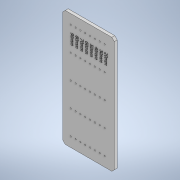
# Autodesk Inventor part: A-01
Saved by Autodesk Inventor 2022 (Build 260153000, 153)
## iProperties
Created: 2021-10-10
Part Number: A-01
Material: Generic
Document SubType Name: Modeling
Designer: kfcs7
Density: 1 g/cm^3
Appearance: Default
Author: kfcs7
Autodesk Inventor part; units mm, degrees
(part 1 of 2)
ref_plane "YZ Plane" through (0, 0, 0) normal (1, 0, 0) x (0, 1, 0)
ref_plane "XZ Plane" through (0, 0, 0) normal (0, 1, 0) x (-1, 0, 0)
ref_plane "XY Plane" through (0, 0, 0) normal (0, 0, 1) x (1, 0, 0)
sketch "Sketch1" plane through (0, 0, 0) normal (0, 0, 1) x (1, 0, 0)
  line L0 (14.5, -5) -> (14.5, -245) construction
  line L1 (14.5, -5) -> (0, -5) construction
  line L2 (0, -5) -> (0, -245) construction
  line L3 (0, -245) -> (14.5, -245) construction
  circle A0 centre (6.5, -25) radius 3.25 construction
  circle A1 centre (6.5, -75) radius 3.25 construction
  circle A2 centre (6.5, -125) radius 3.25 construction
  circle A3 centre (6.5, -175) radius 3.25 construction
  circle A4 centre (6.5, -225) radius 3.25 construction
  line L4 (26.5, -5) -> (-80, -5)
  line L5 (-80, -5) -> (-80, -245)
  line L6 (-80, -245) -> (26.5, -245)
  line L7 (26.5, -245) -> (26.5, -5)
  point P0 (0, 0)
  dimension "d6" = 20
  dimension "d9" = 80
  constraints: 8 end point, 2 collinear, 2 parallel, 1 horizontal, 1 perpendicular
  measures "d6" distance from line of L7 A0.centre
  measures "d9" distance between parallel lines of L2 L5
extrude "Extrusion1" add sketch "Sketch1" along normal blind 6
sketch "Sketch3" plane through (0, 0, 6) normal (0, 0, 1) x (1, 0, 0)
  line L0 (14.5, -5) -> (14.5, -245) construction
  line L1 (14.5, -5) -> (0, -5) construction
  line L2 (0, -5) -> (0, -245) construction
  line L3 (0, -245) -> (14.5, -245) construction
  circle A0 centre (6.5, -25) radius 3.25 construction
  circle A1 centre (6.5, -75) radius 3.25 construction
  circle A2 centre (6.5, -125) radius 3.25 construction
  circle A3 centre (6.5, -175) radius 3.25 construction
  circle A4 centre (6.5, -225) radius 3.25 construction
  circle A5 centre (6.5, -25) radius 1.25
  circle A6 centre (6.5, -75) radius 1.25
  circle A7 centre (6.5, -125) radius 1.25
  circle A8 centre (6.5, -175) radius 1.25
  circle A9 centre (6.5, -225) radius 1.25
  point P0 (0, 0)
  dimension "d10" = 2.5
  dimension "d11" = 2.5
  dimension "d12" = 2.5
  dimension "d13" = 2.5
  dimension "d14" = 2.5
  constraints: 5 centre point, 5 coincident
  measures "d10" diameter of A5
  measures "d11" diameter of A6
  measures "d12" diameter of A7
  measures "d13" diameter of A8
  measures "d14" diameter of A9
extrude "Extrusion2" cut sketch "Sketch3" against normal through all
chamfer "Chamfer1" distance 5 angle 45 4 edges at (26.5, -5, 3) (-80, -5, 3) (-80, -245, 3) (26.5, -245, 3)
pattern_linear "Rectangular Pattern1" count 8 spacing 10 along (-1, 0, 0) of "Extrusion2"
sketch "Sketch4" plane through (0, 0, 6) normal (0, 0, 1) x (1, 0, 0)
  circle A0 centre (6.5, -75) radius 1.25 construction
  circle A1 centre (6.5, -175) radius 1.25 construction
  circle A2 centre (6.5, -125) radius 1.25 construction
  circle A3 centre (6.5, -25) radius 1.25 construction
  circle A4 centre (6.5, -225) radius 1.25 construction
  line L0 (-80, -10) -> (-80, -240) construction
  line L1 (-75, -245) -> (21.5, -245) construction
  line L2 (26.5, -240) -> (26.5, -10) construction
  line L3 (21.5, -5) -> (-75, -5) construction
  circle A5 centre (6.5, -25) radius 1.25 construction
  circle A6 centre (6.5, -75) radius 1.25 construction
  line L4 (6.5, -25) -> (6.5, -75) construction
  line L5 (26.5, -240) -> (21.5, -245) construction
  line L6 (21.5, -5) -> (26.5, -10) construction
  line L7 (-80, -10) -> (-75, -5) construction
  line L8 (-75, -245) -> (-80, -240) construction
  circle A7 centre (-63.5, -75) radius 1.25 construction
  circle A8 centre (-63.5, -225) radius 1.25 construction
  circle A9 centre (-63.5, -25) radius 1.25 construction
  circle A10 centre (-63.5, -125) radius 1.25 construction
  circle A11 centre (-63.5, -175) radius 1.25 construction
  circle A12 centre (-53.5, -75) radius 1.25 construction
  circle A13 centre (-53.5, -225) radius 1.25 construction
  circle A14 centre (-53.5, -25) radius 1.25 construction
  circle A15 centre (-53.5, -125) radius 1.25 construction
  circle A16 centre (-53.5, -175) radius 1.25 construction
  circle A17 centre (-43.5, -75) radius 1.25 construction
  circle A18 centre (-43.5, -225) radius 1.25 construction
  circle A19 centre (-43.5, -25) radius 1.25 construction
  circle A20 centre (-43.5, -125) radius 1.25 construction
  circle A21 centre (-43.5, -175) radius 1.25 construction
  circle A22 centre (-33.5, -75) radius 1.25 construction
  circle A23 centre (-33.5, -225) radius 1.25 construction
  circle A24 centre (-33.5, -25) radius 1.25 construction
  circle A25 centre (-33.5, -125) radius 1.25 construction
  circle A26 centre (-33.5, -175) radius 1.25 construction
  circle A27 centre (-23.5, -75) radius 1.25 construction
  circle A28 centre (-23.5, -225) radius 1.25 construction
  circle A29 centre (-23.5, -25) radius 1.25 construction
  circle A30 centre (-23.5, -125) radius 1.25 construction
  circle A31 centre (-23.5, -175) radius 1.25 construction
  circle A32 centre (-13.5, -75) radius 1.25 construction
  circle A33 centre (-13.5, -225) radius 1.25 construction
  circle A34 centre (-13.5, -25) radius 1.25 construction
  circle A35 centre (-13.5, -125) radius 1.25 construction
  circle A36 centre (-13.5, -175) radius 1.25 construction
  circle A37 centre (-3.5, -75) radius 1.25 construction
  circle A38 centre (-3.5, -225) radius 1.25 construction
  circle A39 centre (-3.5, -25) radius 1.25 construction
  circle A40 centre (-3.5, -125) radius 1.25 construction
  circle A41 centre (-3.5, -175) radius 1.25 construction
  line L9 (26.5, -240) -> (21.5, -245) construction
  line L10 (26.5, -240) -> (26.5, -10) construction
  line L11 (21.5, -5) -> (26.5, -10) construction
  line L12 (21.5, -5) -> (-75, -5) construction
  line L13 (-80, -10) -> (-75, -5) construction
  line L14 (-80, -10) -> (-80, -240) construction
  line L15 (-75, -245) -> (-80, -240) construction
  line L16 (-75, -245) -> (21.5, -245) construction
  circle A42 centre (6.5, -75) radius 1.25 construction
  circle A43 centre (6.5, -175) radius 1.25 construction
  circle A44 centre (6.5, -125) radius 1.25 construction
  circle A45 centre (6.5, -25) radius 1.25 construction
  circle A46 centre (6.5, -225) radius 1.25 construction
  circle A47 centre (-3.5, -25) radius 1.25 construction
  line L17 (-3.5, -25) -> (-3.5, -75) construction
  circle A48 centre (-13.5, -75) radius 1.25 construction
  line L18 (-13.5, -25) -> (-13.5, -75) construction
  circle A49 centre (-23.5, -75) radius 1.25 construction
  circle A50 centre (-23.5, -25) radius 1.25 construction
  line L19 (-23.5, -75) -> (-23.5, -25) construction
  circle A51 centre (-33.5, -25) radius 1.25 construction
  circle A52 centre (-33.5, -75) radius 1.25 construction
  line L20 (-33.5, -25) -> (-33.5, -75) construction
  circle A53 centre (-43.5, -75) radius 1.25 construction
  circle A54 centre (-43.5, -25) radius 1.25 construction
  line L21 (-43.5, -75) -> (-43.5, -25) construction
  circle A55 centre (-53.5, -25) radius 1.25 construction
  circle A56 centre (-53.5, -75) radius 1.25 construction
  line L22 (-53.5, -25) -> (-53.5, -75) construction
  circle A57 centre (-63.5, -25) radius 1.25 construction
  circle A58 centre (-63.5, -75) radius 1.25 construction
  line L23 (-63.5, -25) -> (-63.5, -75) construction
  line L24 (6.5, -42.5851) -> (6.5, -38.8233)
  line L25 (6.5, -38.8233) -> (7.3651, -38.8233)
  spline S0 degree 2 poles (7.3651, -38.8233) (7.7457, -39.2286) (8.4526, -39.9503) (8.8332, -40.2964) knots 0 0 0 1 2 2 2
  spline S1 degree 2 poles (8.8332, -40.2964) (9.5994, -40.9934) (10.5189, -41.5025) (11.0083, -41.5025) knots 0 0 0 1 2 2 2
  spline S2 degree 2 poles (11.0083, -41.5025) (11.2653, -41.5025) (11.6509, -41.3443) (11.7745, -41.201) knots 0 0 0 1 2 2 2
  spline S3 degree 2 poles (11.7745, -41.201) (11.8981, -41.0576) (12.0216, -40.6819) (12.0216, -40.4545) knots 0 0 0 1 2 2 2
  spline S4 degree 2 poles (12.0216, -40.4545) (12.0216, -40.237) (11.9129, -39.7921) (11.8288, -39.5895) knots 0 0 0 1 2 2 2
  spline S5 degree 2 poles (11.8288, -39.5895) (11.7596, -39.4165) (11.5619, -39.0951) (11.4927, -38.9963) knots 0 0 0 1 2 2 2
  line L26 (11.4927, -38.9963) -> (11.4927, -38.9518)
  line L27 (11.4927, -38.9518) -> (12.3627, -38.9518)
  spline S6 degree 2 poles (12.3627, -38.9518) (12.4863, -39.2039) (12.7285, -40.1085) (12.7285, -40.5139) knots 0 0 0 1 2 2 2
  spline S7 degree 2 poles (12.7285, -40.5139) (12.7285, -41.369) (11.8239, -42.333) (11.0528, -42.333) knots 0 0 0 1 2 2 2
  spline S8 degree 2 poles (11.0528, -42.333) (10.6919, -42.333) (10.0888, -42.1649) (9.8318, -42.0166) knots 0 0 0 1 2 2 2
  spline S9 degree 2 poles (9.8318, -42.0166) (9.5648, -41.8683) (9.0408, -41.4382) (8.7887, -41.201) knots 0 0 0 1 2 2 2
  spline S10 degree 2 poles (8.7887, -41.201) (8.3686, -40.8154) (7.4689, -39.8712) (7.2069, -39.5895) knots 0 0 0 1 2 2 2
  line L28 (7.2069, -39.5895) -> (7.2069, -42.5851)
  line L29 (7.2069, -42.5851) -> (6.5, -42.5851)
  spline S11 degree 2 poles (9.55, -47.1972) (7.9088, -47.1972) (6.3715, -46.2431) (6.3715, -45.2495) knots 0 0 0 1 2 2 2
  spline S12 degree 2 poles (6.3715, -45.2495) (6.3715, -44.2411) (7.9385, -43.2969) (9.5451, -43.2969) knots 0 0 0 1 2 2 2
  spline S13 degree 2 poles (9.5451, -43.2969) (11.1961, -43.2969) (12.7236, -44.251) (12.7236, -45.2495) knots 0 0 0 1 2 2 2
  spline S14 degree 2 poles (12.7236, -45.2495) (12.7236, -46.253) (11.1417, -47.1972) (9.55, -47.1972) knots 0 0 0 1 2 2 2
  spline S15 degree 2 poles (7.6913, -46.1492) (7.9929, -46.2678) (8.9222, -46.3667) (9.55, -46.3667) knots 0 0 0 1 2 2 2
  spline S16 degree 2 poles (9.55, -46.3667) (10.1778, -46.3667) (11.1022, -46.2678) (11.4136, -46.1442) knots 0 0 0 1 2 2 2
  spline S17 degree 2 poles (11.4136, -46.1442) (11.725, -46.0207) (12.0464, -45.5906) (12.0464, -45.2495) knots 0 0 0 1 2 2 2
  spline S18 degree 2 poles (12.0464, -45.2495) (12.0464, -44.9084) (11.725, -44.4685) (11.4037, -44.34) knots 0 0 0 1 2 2 2
  spline S19 degree 2 poles (11.4037, -44.34) (11.0923, -44.2164) (10.1432, -44.1274) (9.5451, -44.1274) knots 0 0 0 1 2 2 2
  spline S20 degree 2 poles (9.5451, -44.1274) (8.9024, -44.1274) (8.0423, -44.2065) (7.7062, -44.335) knots 0 0 0 1 2 2 2
  spline S21 degree 2 poles (7.7062, -44.335) (7.3898, -44.4536) (7.0487, -44.8936) (7.0487, -45.2495) knots 0 0 0 1 2 2 2
  spline S22 degree 2 poles (7.0487, -45.2495) (7.0487, -45.5857) (7.37, -46.0256) (7.6913, -46.1492) knots 0 0 0 1 2 2 2
  line L30 (6.5, -53.2823) -> (9.1496, -53.2823)
  spline S23 degree 2 poles (9.1496, -53.2823) (9.466, -53.2823) (10.0048, -53.2329) (10.1531, -53.1538) knots 0 0 0 1 2 2 2
  spline S24 degree 2 poles (10.1531, -53.1538) (10.3162, -53.0747) (10.4744, -52.7732) (10.4744, -52.5112) knots 0 0 0 1 2 2 2
  spline S25 degree 2 poles (10.4744, -52.5112) (10.4744, -52.2739) (10.1827, -51.7301) (9.9059, -51.4434) knots 0 0 0 1 2 2 2
  spline S26 degree 2 poles (9.9059, -51.4434) (9.8367, -51.4484) (9.6439, -51.4583) (9.5154, -51.4583) knots 0 0 0 1 2 2 2
  line L31 (9.5154, -51.4583) -> (6.5, -51.4583)
  line L32 (6.5, -51.4583) -> (6.5, -50.6871)
  line L33 (6.5, -50.6871) -> (9.1496, -50.6871)
  spline S27 degree 2 poles (9.1496, -50.6871) (9.466, -50.6871) (10.0048, -50.6377) (10.1531, -50.5586) knots 0 0 0 1 2 2 2
  spline S28 degree 2 poles (10.1531, -50.5586) (10.3162, -50.4795) (10.4744, -50.178) (10.4744, -49.916) knots 0 0 0 1 2 2 2
  spline S29 degree 2 poles (10.4744, -49.916) (10.4744, -49.6688) (10.163, -49.1201) (9.9207, -48.863) knots 0 0 0 1 2 2 2
  line L34 (9.9207, -48.863) -> (6.5, -48.863)
  line L35 (6.5, -48.863) -> (6.5, -48.0919)
  line L36 (6.5, -48.0919) -> (11.0775, -48.0919)
  line L37 (11.0775, -48.0919) -> (11.0775, -48.863)
  line L38 (11.0775, -48.863) -> (10.5733, -48.863)
  spline S30 degree 2 poles (10.5733, -48.863) (10.8748, -49.1646) (11.206, -49.7578) (11.206, -50.1137) knots 0 0 0 1 2 2 2
  spline S31 degree 2 poles (11.206, -50.1137) (11.206, -50.519) (10.8353, -51.1468) (10.4151, -51.31) knots 0 0 0 1 2 2 2
  spline S32 degree 2 poles (10.4151, -51.31) (10.8056, -51.6609) (11.206, -52.3233) (11.206, -52.7089) knots 0 0 0 1 2 2 2
  spline S33 degree 2 poles (11.206, -52.7089) (11.206, -53.0055) (11.0231, -53.49) (10.8155, -53.6679) knots 0 0 0 1 2 2 2
  spline S34 degree 2 poles (10.8155, -53.6679) (10.6079, -53.8508) (9.985, -54.0535) (9.5154, -54.0535) knots 0 0 0 1 2 2 2
  line L39 (9.5154, -54.0535) -> (6.5, -54.0535)
  line L40 (6.5, -54.0535) -> (6.5, -53.2823)
  line L41 (6.5, -60.3265) -> (9.1496, -60.3265)
  spline S35 degree 2 poles (9.1496, -60.3265) (9.466, -60.3265) (10.0048, -60.2771) (10.1531, -60.198) knots 0 0 0 1 2 2 2
  spline S36 degree 2 poles (10.1531, -60.198) (10.3162, -60.1189) (10.4744, -59.8173) (10.4744, -59.5553) knots 0 0 0 1 2 2 2
  spline S37 degree 2 poles (10.4744, -59.5553) (10.4744, -59.3181) (10.1827, -58.7743) (9.9059, -58.4876) knots 0 0 0 1 2 2 2
  spline S38 degree 2 poles (9.9059, -58.4876) (9.8367, -58.4925) (9.6439, -58.5024) (9.5154, -58.5024) knots 0 0 0 1 2 2 2
  line L42 (9.5154, -58.5024) -> (6.5, -58.5024)
  line L43 (6.5, -58.5024) -> (6.5, -57.7313)
  line L44 (6.5, -57.7313) -> (9.1496, -57.7313)
  spline S39 degree 2 poles (9.1496, -57.7313) (9.466, -57.7313) (10.0048, -57.6818) (10.1531, -57.6028) knots 0 0 0 1 2 2 2
  spline S40 degree 2 poles (10.1531, -57.6028) (10.3162, -57.5237) (10.4744, -57.2221) (10.4744, -56.9601) knots 0 0 0 1 2 2 2
  spline S41 degree 2 poles (10.4744, -56.9601) (10.4744, -56.713) (10.163, -56.1643) (9.9207, -55.9072) knots 0 0 0 1 2 2 2
  line L45 (9.9207, -55.9072) -> (6.5, -55.9072)
  line L46 (6.5, -55.9072) -> (6.5, -55.1361)
  line L47 (6.5, -55.1361) -> (11.0775, -55.1361)
  line L48 (11.0775, -55.1361) -> (11.0775, -55.9072)
  line L49 (11.0775, -55.9072) -> (10.5733, -55.9072)
  spline S42 degree 2 poles (10.5733, -55.9072) (10.8748, -56.2088) (11.206, -56.8019) (11.206, -57.1579) knots 0 0 0 1 2 2 2
  spline S43 degree 2 poles (11.206, -57.1579) (11.206, -57.5632) (10.8353, -58.191) (10.4151, -58.3541) knots 0 0 0 1 2 2 2
  spline S44 degree 2 poles (10.4151, -58.3541) (10.8056, -58.7051) (11.206, -59.3675) (11.206, -59.7531) knots 0 0 0 1 2 2 2
  spline S45 degree 2 poles (11.206, -59.7531) (11.206, -60.0497) (11.0231, -60.5341) (10.8155, -60.7121) knots 0 0 0 1 2 2 2
  spline S46 degree 2 poles (10.8155, -60.7121) (10.6079, -60.895) (9.985, -61.0976) (9.5154, -61.0976) knots 0 0 0 1 2 2 2
  line L50 (9.5154, -61.0976) -> (6.5, -61.0976)
  line L51 (6.5, -61.0976) -> (6.5, -60.3265)
  spline S47 degree 2 poles (2.0216, -40.4694) (2.0216, -40.2469) (1.9129, -39.807) (1.8288, -39.5944) knots 0 0 0 1 2 2 2
  spline S48 degree 2 poles (1.8288, -39.5944) (1.7448, -39.3967) (1.5669, -39.105) (1.4878, -38.9913) knots 0 0 0 1 2 2 2
  line L52 (1.4878, -38.9913) -> (1.4878, -38.9419)
  line L53 (1.4878, -38.9419) -> (2.3528, -38.9419)
  spline S49 degree 2 poles (2.3528, -38.9419) (2.4962, -39.2088) (2.7285, -40.1233) (2.7285, -40.5336) knots 0 0 0 1 2 2 2
  spline S50 degree 2 poles (2.7285, -40.5336) (2.7285, -40.9489) (2.5605, -41.5668) (2.3825, -41.8189) knots 0 0 0 1 2 2 2
  spline S51 degree 2 poles (2.3825, -41.8189) (2.1897, -42.0858) (1.6311, -42.3626) (1.2554, -42.3626) knots 0 0 0 1 2 2 2
  spline S52 degree 2 poles (1.2554, -42.3626) (0.7512, -42.3626) (-0.01, -41.7002) (-0.1089, -41.2356) knots 0 0 0 1 2 2 2
  line L54 (-0.1089, -41.2356) -> (-0.1682, -41.2356)
  spline S53 degree 2 poles (-0.1682, -41.2356) (-0.2078, -41.4284) (-0.3857, -41.8683) (-0.5637, -42.0562) knots 0 0 0 1 2 2 2
  spline S54 degree 2 poles (-0.5637, -42.0562) (-0.7367, -42.244) (-1.2904, -42.4813) (-1.6908, -42.4813) knots 0 0 0 1 2 2 2
  spline S55 degree 2 poles (-1.6908, -42.4813) (-2.1011, -42.4813) (-2.7981, -42.1995) (-3.065, -41.9425) knots 0 0 0 1 2 2 2
  spline S56 degree 2 poles (-3.065, -41.9425) (-3.3418, -41.6755) (-3.6285, -40.9192) (-3.6285, -40.4397) knots 0 0 0 1 2 2 2
  spline S57 degree 2 poles (-3.6285, -40.4397) (-3.6285, -39.98) (-3.4061, -39.0803) (-3.2528, -38.7738) knots 0 0 0 1 2 2 2
  line L55 (-3.2528, -38.7738) -> (-2.3878, -38.7738)
  line L56 (-2.3878, -38.7738) -> (-2.3878, -38.8331)
  spline S58 degree 2 poles (-2.3878, -38.8331) (-2.5756, -39.0902) (-2.9216, -39.9602) (-2.9216, -40.3903) knots 0 0 0 1 2 2 2
  spline S59 degree 2 poles (-2.9216, -40.3903) (-2.9216, -40.6424) (-2.7635, -41.1466) (-2.5806, -41.3147) knots 0 0 0 1 2 2 2
  spline S60 degree 2 poles (-2.5806, -41.3147) (-2.3976, -41.4778) (-1.9626, -41.6508) (-1.6314, -41.6508) knots 0 0 0 1 2 2 2
  spline S61 degree 2 poles (-1.6314, -41.6508) (-1.3002, -41.6508) (-0.8702, -41.458) (-0.7466, -41.285) knots 0 0 0 1 2 2 2
  spline S62 degree 2 poles (-0.7466, -41.285) (-0.623, -41.112) (-0.5291, -40.6424) (-0.5291, -40.3656) knots 0 0 0 1 2 2 2
  line L57 (-0.5291, -40.3656) -> (-0.5291, -40.0195)
  line L58 (-0.5291, -40.0195) -> (0.1481, -40.0195)
  line L59 (0.1481, -40.0195) -> (0.1481, -40.2914)
  spline S63 degree 2 poles (0.1481, -40.2914) (0.1481, -40.8401) (0.6721, -41.5322) (1.1714, -41.5322) knots 0 0 0 1 2 2 2
  spline S64 degree 2 poles (1.1714, -41.5322) (1.4037, -41.5322) (1.7349, -41.3542) (1.8338, -41.2109) knots 0 0 0 1 2 2 2
  spline S65 degree 2 poles (1.8338, -41.2109) (1.9376, -41.0576) (2.0216, -40.6819) (2.0216, -40.4694) knots 0 0 0 1 2 2 2
  spline S66 degree 2 poles (-0.45, -47.1972) (-2.0912, -47.1972) (-3.6285, -46.2431) (-3.6285, -45.2495) knots 0 0 0 1 2 2 2
  spline S67 degree 2 poles (-3.6285, -45.2495) (-3.6285, -44.2411) (-2.0615, -43.2969) (-0.4549, -43.2969) knots 0 0 0 1 2 2 2
  spline S68 degree 2 poles (-0.4549, -43.2969) (1.1961, -43.2969) (2.7236, -44.251) (2.7236, -45.2495) knots 0 0 0 1 2 2 2
  spline S69 degree 2 poles (2.7236, -45.2495) (2.7236, -46.253) (1.1417, -47.1972) (-0.45, -47.1972) knots 0 0 0 1 2 2 2
  spline S70 degree 2 poles (-2.3087, -46.1492) (-2.0071, -46.2678) (-1.0778, -46.3667) (-0.45, -46.3667) knots 0 0 0 1 2 2 2
  spline S71 degree 2 poles (-0.45, -46.3667) (0.1778, -46.3667) (1.1022, -46.2678) (1.4136, -46.1442) knots 0 0 0 1 2 2 2
  spline S72 degree 2 poles (1.4136, -46.1442) (1.725, -46.0207) (2.0464, -45.5906) (2.0464, -45.2495) knots 0 0 0 1 2 2 2
  spline S73 degree 2 poles (2.0464, -45.2495) (2.0464, -44.9084) (1.725, -44.4685) (1.4037, -44.34) knots 0 0 0 1 2 2 2
  spline S74 degree 2 poles (1.4037, -44.34) (1.0923, -44.2164) (0.1432, -44.1274) (-0.4549, -44.1274) knots 0 0 0 1 2 2 2
  spline S75 degree 2 poles (-0.4549, -44.1274) (-1.0976, -44.1274) (-1.9577, -44.2065) (-2.2938, -44.335) knots 0 0 0 1 2 2 2
  spline S76 degree 2 poles (-2.2938, -44.335) (-2.6102, -44.4536) (-2.9513, -44.8936) (-2.9513, -45.2495) knots 0 0 0 1 2 2 2
  spline S77 degree 2 poles (-2.9513, -45.2495) (-2.9513, -45.5857) (-2.63, -46.0256) (-2.3087, -46.1492) knots 0 0 0 1 2 2 2
  line L60 (-3.5, -53.2823) -> (-0.8504, -53.2823)
  spline S78 degree 2 poles (-0.8504, -53.2823) (-0.534, -53.2823) (0.0048, -53.2329) (0.1531, -53.1538) knots 0 0 0 1 2 2 2
  spline S79 degree 2 poles (0.1531, -53.1538) (0.3162, -53.0747) (0.4744, -52.7732) (0.4744, -52.5112) knots 0 0 0 1 2 2 2
  spline S80 degree 2 poles (0.4744, -52.5112) (0.4744, -52.2739) (0.1827, -51.7301) (-0.0941, -51.4434) knots 0 0 0 1 2 2 2
  spline S81 degree 2 poles (-0.0941, -51.4434) (-0.1633, -51.4484) (-0.3561, -51.4583) (-0.4846, -51.4583) knots 0 0 0 1 2 2 2
  line L61 (-0.4846, -51.4583) -> (-3.5, -51.4583)
  line L62 (-3.5, -51.4583) -> (-3.5, -50.6871)
  line L63 (-3.5, -50.6871) -> (-0.8504, -50.6871)
  spline S82 degree 2 poles (-0.8504, -50.6871) (-0.534, -50.6871) (0.0048, -50.6377) (0.1531, -50.5586) knots 0 0 0 1 2 2 2
  spline S83 degree 2 poles (0.1531, -50.5586) (0.3162, -50.4795) (0.4744, -50.178) (0.4744, -49.916) knots 0 0 0 1 2 2 2
  spline S84 degree 2 poles (0.4744, -49.916) (0.4744, -49.6688) (0.163, -49.1201) (-0.0793, -48.863) knots 0 0 0 1 2 2 2
  line L64 (-0.0793, -48.863) -> (-3.5, -48.863)
  line L65 (-3.5, -48.863) -> (-3.5, -48.0919)
  line L66 (-3.5, -48.0919) -> (1.0775, -48.0919)
  line L67 (1.0775, -48.0919) -> (1.0775, -48.863)
  line L68 (1.0775, -48.863) -> (0.5733, -48.863)
  spline S85 degree 2 poles (0.5733, -48.863) (0.8748, -49.1646) (1.206, -49.7578) (1.206, -50.1137) knots 0 0 0 1 2 2 2
  spline S86 degree 2 poles (1.206, -50.1137) (1.206, -50.519) (0.8353, -51.1468) (0.4151, -51.31) knots 0 0 0 1 2 2 2
  spline S87 degree 2 poles (0.4151, -51.31) (0.8056, -51.6609) (1.206, -52.3233) (1.206, -52.7089) knots 0 0 0 1 2 2 2
  spline S88 degree 2 poles (1.206, -52.7089) (1.206, -53.0055) (1.0231, -53.49) (0.8155, -53.6679) knots 0 0 0 1 2 2 2
  spline S89 degree 2 poles (0.8155, -53.6679) (0.6079, -53.8508) (-0.015, -54.0535) (-0.4846, -54.0535) knots 0 0 0 1 2 2 2
  line L69 (-0.4846, -54.0535) -> (-3.5, -54.0535)
  line L70 (-3.5, -54.0535) -> (-3.5, -53.2823)
  line L71 (-3.5, -60.3265) -> (-0.8504, -60.3265)
  spline S90 degree 2 poles (-0.8504, -60.3265) (-0.534, -60.3265) (0.0048, -60.2771) (0.1531, -60.198) knots 0 0 0 1 2 2 2
  spline S91 degree 2 poles (0.1531, -60.198) (0.3162, -60.1189) (0.4744, -59.8173) (0.4744, -59.5553) knots 0 0 0 1 2 2 2
  spline S92 degree 2 poles (0.4744, -59.5553) (0.4744, -59.3181) (0.1827, -58.7743) (-0.0941, -58.4876) knots 0 0 0 1 2 2 2
  spline S93 degree 2 poles (-0.0941, -58.4876) (-0.1633, -58.4925) (-0.3561, -58.5024) (-0.4846, -58.5024) knots 0 0 0 1 2 2 2
  line L72 (-0.4846, -58.5024) -> (-3.5, -58.5024)
  line L73 (-3.5, -58.5024) -> (-3.5, -57.7313)
  line L74 (-3.5, -57.7313) -> (-0.8504, -57.7313)
  spline S94 degree 2 poles (-0.8504, -57.7313) (-0.534, -57.7313) (0.0048, -57.6818) (0.1531, -57.6028) knots 0 0 0 1 2 2 2
  spline S95 degree 2 poles (0.1531, -57.6028) (0.3162, -57.5237) (0.4744, -57.2221) (0.4744, -56.9601) knots 0 0 0 1 2 2 2
  spline S96 degree 2 poles (0.4744, -56.9601) (0.4744, -56.713) (0.163, -56.1643) (-0.0793, -55.9072) knots 0 0 0 1 2 2 2
  line L75 (-0.0793, -55.9072) -> (-3.5, -55.9072)
  line L76 (-3.5, -55.9072) -> (-3.5, -55.1361)
  line L77 (-3.5, -55.1361) -> (1.0775, -55.1361)
  line L78 (1.0775, -55.1361) -> (1.0775, -55.9072)
  line L79 (1.0775, -55.9072) -> (0.5733, -55.9072)
  spline S97 degree 2 poles (0.5733, -55.9072) (0.8748, -56.2088) (1.206, -56.8019) (1.206, -57.1579) knots 0 0 0 1 2 2 2
  spline S98 degree 2 poles (1.206, -57.1579) (1.206, -57.5632) (0.8353, -58.191) (0.4151, -58.3541) knots 0 0 0 1 2 2 2
  spline S99 degree 2 poles (0.4151, -58.3541) (0.8056, -58.7051) (1.206, -59.3675) (1.206, -59.7531) knots 0 0 0 1 2 2 2
  spline S100 degree 2 poles (1.206, -59.7531) (1.206, -60.0497) (1.0231, -60.5341) (0.8155, -60.7121) knots 0 0 0 1 2 2 2
  spline S101 degree 2 poles (0.8155, -60.7121) (0.6079, -60.895) (-0.015, -61.0976) (-0.4846, -61.0976) knots 0 0 0 1 2 2 2
  line L80 (-0.4846, -61.0976) -> (-3.5, -61.0976)
  line L81 (-3.5, -61.0976) -> (-3.5, -60.3265)
  line L82 (-11.4041, -42.7482) -> (-11.4041, -42.0216)
  line L83 (-11.4041, -42.0216) -> (-13.5, -42.0216)
  line L84 (-13.5, -42.0216) -> (-13.5, -41.2356)
  line L85 (-13.5, -41.2356) -> (-11.4041, -41.2356)
  line L86 (-11.4041, -41.2356) -> (-11.4041, -38.5415)
  line L87 (-11.4041, -38.5415) -> (-10.5439, -38.5415)
  line L88 (-10.5439, -38.5415) -> (-7.4, -41.2702)
  line L89 (-7.4, -41.2702) -> (-7.4, -42.0216)
  line L90 (-7.4, -42.0216) -> (-10.7466, -42.0216)
  line L91 (-10.7466, -42.0216) -> (-10.7466, -42.7482)
  line L92 (-10.7466, -42.7482) -> (-11.4041, -42.7482)
  line L93 (-10.7466, -41.2356) -> (-8.3639, -41.2356)
  line L94 (-8.3639, -41.2356) -> (-10.7466, -39.1841)
  line L95 (-10.7466, -39.1841) -> (-10.7466, -41.2356)
  spline S102 degree 2 poles (-10.45, -47.1972) (-12.0912, -47.1972) (-13.6285, -46.2431) (-13.6285, -45.2495) knots 0 0 0 1 2 2 2
  spline S103 degree 2 poles (-13.6285, -45.2495) (-13.6285, -44.2411) (-12.0615, -43.2969) (-10.4549, -43.2969) knots 0 0 0 1 2 2 2
  spline S104 degree 2 poles (-10.4549, -43.2969) (-8.8039, -43.2969) (-7.2764, -44.251) (-7.2764, -45.2495) knots 0 0 0 1 2 2 2
  spline S105 degree 2 poles (-7.2764, -45.2495) (-7.2764, -46.253) (-8.8583, -47.1972) (-10.45, -47.1972) knots 0 0 0 1 2 2 2
  spline S106 degree 2 poles (-12.3087, -46.1492) (-12.0071, -46.2678) (-11.0778, -46.3667) (-10.45, -46.3667) knots 0 0 0 1 2 2 2
  spline S107 degree 2 poles (-10.45, -46.3667) (-9.8222, -46.3667) (-8.8978, -46.2678) (-8.5864, -46.1442) knots 0 0 0 1 2 2 2
  spline S108 degree 2 poles (-8.5864, -46.1442) (-8.275, -46.0207) (-7.9536, -45.5906) (-7.9536, -45.2495) knots 0 0 0 1 2 2 2
  spline S109 degree 2 poles (-7.9536, -45.2495) (-7.9536, -44.9084) (-8.275, -44.4685) (-8.5963, -44.34) knots 0 0 0 1 2 2 2
  spline S110 degree 2 poles (-8.5963, -44.34) (-8.9077, -44.2164) (-9.8568, -44.1274) (-10.4549, -44.1274) knots 0 0 0 1 2 2 2
  spline S111 degree 2 poles (-10.4549, -44.1274) (-11.0976, -44.1274) (-11.9577, -44.2065) (-12.2938, -44.335) knots 0 0 0 1 2 2 2
  spline S112 degree 2 poles (-12.2938, -44.335) (-12.6102, -44.4536) (-12.9513, -44.8936) (-12.9513, -45.2495) knots 0 0 0 1 2 2 2
  spline S113 degree 2 poles (-12.9513, -45.2495) (-12.9513, -45.5857) (-12.63, -46.0256) (-12.3087, -46.1492) knots 0 0 0 1 2 2 2
  line L96 (-13.5, -53.2823) -> (-10.8504, -53.2823)
  spline S114 degree 2 poles (-10.8504, -53.2823) (-10.534, -53.2823) (-9.9952, -53.2329) (-9.8469, -53.1538) knots 0 0 0 1 2 2 2
  spline S115 degree 2 poles (-9.8469, -53.1538) (-9.6838, -53.0747) (-9.5256, -52.7732) (-9.5256, -52.5112) knots 0 0 0 1 2 2 2
  spline S116 degree 2 poles (-9.5256, -52.5112) (-9.5256, -52.2739) (-9.8173, -51.7301) (-10.0941, -51.4434) knots 0 0 0 1 2 2 2
  spline S117 degree 2 poles (-10.0941, -51.4434) (-10.1633, -51.4484) (-10.3561, -51.4583) (-10.4846, -51.4583) knots 0 0 0 1 2 2 2
  line L97 (-10.4846, -51.4583) -> (-13.5, -51.4583)
  line L98 (-13.5, -51.4583) -> (-13.5, -50.6871)
  line L99 (-13.5, -50.6871) -> (-10.8504, -50.6871)
  spline S118 degree 2 poles (-10.8504, -50.6871) (-10.534, -50.6871) (-9.9952, -50.6377) (-9.8469, -50.5586) knots 0 0 0 1 2 2 2
  spline S119 degree 2 poles (-9.8469, -50.5586) (-9.6838, -50.4795) (-9.5256, -50.178) (-9.5256, -49.916) knots 0 0 0 1 2 2 2
  spline S120 degree 2 poles (-9.5256, -49.916) (-9.5256, -49.6688) (-9.837, -49.1201) (-10.0793, -48.863) knots 0 0 0 1 2 2 2
  line L100 (-10.0793, -48.863) -> (-13.5, -48.863)
  line L101 (-13.5, -48.863) -> (-13.5, -48.0919)
  line L102 (-13.5, -48.0919) -> (-8.9225, -48.0919)
  line L103 (-8.9225, -48.0919) -> (-8.9225, -48.863)
  line L104 (-8.9225, -48.863) -> (-9.4267, -48.863)
  spline S121 degree 2 poles (-9.4267, -48.863) (-9.1252, -49.1646) (-8.794, -49.7578) (-8.794, -50.1137) knots 0 0 0 1 2 2 2
  spline S122 degree 2 poles (-8.794, -50.1137) (-8.794, -50.519) (-9.1647, -51.1468) (-9.5849, -51.31) knots 0 0 0 1 2 2 2
  spline S123 degree 2 poles (-9.5849, -51.31) (-9.1944, -51.6609) (-8.794, -52.3233) (-8.794, -52.7089) knots 0 0 0 1 2 2 2
  spline S124 degree 2 poles (-8.794, -52.7089) (-8.794, -53.0055) (-8.9769, -53.49) (-9.1845, -53.6679) knots 0 0 0 1 2 2 2
  spline S125 degree 2 poles (-9.1845, -53.6679) (-9.3921, -53.8508) (-10.015, -54.0535) (-10.4846, -54.0535) knots 0 0 0 1 2 2 2
  line L105 (-10.4846, -54.0535) -> (-13.5, -54.0535)
  line L106 (-13.5, -54.0535) -> (-13.5, -53.2823)
  line L107 (-13.5, -60.3265) -> (-10.8504, -60.3265)
  spline S126 degree 2 poles (-10.8504, -60.3265) (-10.534, -60.3265) (-9.9952, -60.2771) (-9.8469, -60.198) knots 0 0 0 1 2 2 2
  spline S127 degree 2 poles (-9.8469, -60.198) (-9.6838, -60.1189) (-9.5256, -59.8173) (-9.5256, -59.5553) knots 0 0 0 1 2 2 2
  spline S128 degree 2 poles (-9.5256, -59.5553) (-9.5256, -59.3181) (-9.8173, -58.7743) (-10.0941, -58.4876) knots 0 0 0 1 2 2 2
  spline S129 degree 2 poles (-10.0941, -58.4876) (-10.1633, -58.4925) (-10.3561, -58.5024) (-10.4846, -58.5024) knots 0 0 0 1 2 2 2
  line L108 (-10.4846, -58.5024) -> (-13.5, -58.5024)
  line L109 (-13.5, -58.5024) -> (-13.5, -57.7313)
  line L110 (-13.5, -57.7313) -> (-10.8504, -57.7313)
  spline S130 degree 2 poles (-10.8504, -57.7313) (-10.534, -57.7313) (-9.9952, -57.6818) (-9.8469, -57.6028) knots 0 0 0 1 2 2 2
  spline S131 degree 2 poles (-9.8469, -57.6028) (-9.6838, -57.5237) (-9.5256, -57.2221) (-9.5256, -56.9601) knots 0 0 0 1 2 2 2
  spline S132 degree 2 poles (-9.5256, -56.9601) (-9.5256, -56.713) (-9.837, -56.1643) (-10.0793, -55.9072) knots 0 0 0 1 2 2 2
  line L111 (-10.0793, -55.9072) -> (-13.5, -55.9072)
  line L112 (-13.5, -55.9072) -> (-13.5, -55.1361)
  line L113 (-13.5, -55.1361) -> (-8.9225, -55.1361)
  line L114 (-8.9225, -55.1361) -> (-8.9225, -55.9072)
  line L115 (-8.9225, -55.9072) -> (-9.4267, -55.9072)
  spline S133 degree 2 poles (-9.4267, -55.9072) (-9.1252, -56.2088) (-8.794, -56.8019) (-8.794, -57.1579) knots 0 0 0 1 2 2 2
  spline S134 degree 2 poles (-8.794, -57.1579) (-8.794, -57.5632) (-9.1647, -58.191) (-9.5849, -58.3541) knots 0 0 0 1 2 2 2
  spline S135 degree 2 poles (-9.5849, -58.3541) (-9.1944, -58.7051) (-8.794, -59.3675) (-8.794, -59.7531) knots 0 0 0 1 2 2 2
  spline S136 degree 2 poles (-8.794, -59.7531) (-8.794, -60.0497) (-8.9769, -60.5341) (-9.1845, -60.7121) knots 0 0 0 1 2 2 2
  spline S137 degree 2 poles (-9.1845, -60.7121) (-9.3921, -60.895) (-10.015, -61.0976) (-10.4846, -61.0976) knots 0 0 0 1 2 2 2
  line L116 (-10.4846, -61.0976) -> (-13.5, -61.0976)
  line L117 (-13.5, -61.0976) -> (-13.5, -60.3265)
  spline S138 degree 2 poles (-21.5622, -42.5208) (-22.0022, -42.5208) (-22.7536, -42.2391) (-23.0304, -41.982) knots 0 0 0 1 2 2 2
  spline S139 degree 2 poles (-23.0304, -41.982) (-23.3072, -41.725) (-23.6285, -40.9588) (-23.6285, -40.4842) knots 0 0 0 1 2 2 2
  spline S140 degree 2 poles (-23.6285, -40.4842) (-23.6285, -40.0492) (-23.4357, -39.1989) (-23.2825, -38.8875) knots 0 0 0 1 2 2 2
  line L118 (-23.2825, -38.8875) -> (-22.4174, -38.8875)
  line L119 (-22.4174, -38.8875) -> (-22.4174, -38.9468)
  spline S141 degree 2 poles (-22.4174, -38.9468) (-22.4866, -39.0408) (-22.6646, -39.3917) (-22.7437, -39.6043) knots 0 0 0 1 2 2 2
  spline S142 degree 2 poles (-22.7437, -39.6043) (-22.8277, -39.8465) (-22.9216, -40.2469) (-22.9216, -40.499) knots 0 0 0 1 2 2 2
  spline S143 degree 2 poles (-22.9216, -40.499) (-22.9216, -40.7462) (-22.7437, -41.2109) (-22.5509, -41.3789) knots 0 0 0 1 2 2 2
  spline S144 degree 2 poles (-22.5509, -41.3789) (-22.368, -41.5322) (-21.8835, -41.6904) (-21.5573, -41.6904) knots 0 0 0 1 2 2 2
  spline S145 degree 2 poles (-21.5573, -41.6904) (-21.231, -41.6904) (-20.8158, -41.5124) (-20.6774, -41.3443) knots 0 0 0 1 2 2 2
  spline S146 degree 2 poles (-20.6774, -41.3443) (-20.5241, -41.1713) (-20.3956, -40.6572) (-20.3956, -40.3458) knots 0 0 0 1 2 2 2
  spline S147 degree 2 poles (-20.3956, -40.3458) (-20.3956, -40.0096) (-20.4994, -39.3423) (-20.5439, -39.1396) knots 0 0 0 1 2 2 2
  line L120 (-20.5439, -39.1396) -> (-17.4, -39.1396)
  line L121 (-17.4, -39.1396) -> (-17.4, -42.4862)
  line L122 (-17.4, -42.4862) -> (-18.1168, -42.4862)
  line L123 (-18.1168, -42.4862) -> (-18.1168, -39.9256)
  line L124 (-18.1168, -39.9256) -> (-19.7431, -39.9256)
  spline S148 degree 2 poles (-19.7431, -39.9256) (-19.7233, -40.0739) (-19.7085, -40.3606) (-19.7085, -40.4793) knots 0 0 0 1 2 2 2
  spline S149 degree 2 poles (-19.7085, -40.4793) (-19.7085, -40.9489) (-19.8618, -41.5964) (-20.0891, -41.893) knots 0 0 0 1 2 2 2
  spline S150 degree 2 poles (-20.0891, -41.893) (-20.3165, -42.1946) (-21.0086, -42.5208) (-21.5622, -42.5208) knots 0 0 0 1 2 2 2
  spline S151 degree 2 poles (-20.45, -47.1972) (-22.0912, -47.1972) (-23.6285, -46.2431) (-23.6285, -45.2495) knots 0 0 0 1 2 2 2
  spline S152 degree 2 poles (-23.6285, -45.2495) (-23.6285, -44.2411) (-22.0615, -43.2969) (-20.4549, -43.2969) knots 0 0 0 1 2 2 2
  spline S153 degree 2 poles (-20.4549, -43.2969) (-18.8039, -43.2969) (-17.2764, -44.251) (-17.2764, -45.2495) knots 0 0 0 1 2 2 2
  spline S154 degree 2 poles (-17.2764, -45.2495) (-17.2764, -46.253) (-18.8583, -47.1972) (-20.45, -47.1972) knots 0 0 0 1 2 2 2
  spline S155 degree 2 poles (-22.3087, -46.1492) (-22.0071, -46.2678) (-21.0778, -46.3667) (-20.45, -46.3667) knots 0 0 0 1 2 2 2
  spline S156 degree 2 poles (-20.45, -46.3667) (-19.8222, -46.3667) (-18.8978, -46.2678) (-18.5864, -46.1442) knots 0 0 0 1 2 2 2
  spline S157 degree 2 poles (-18.5864, -46.1442) (-18.275, -46.0207) (-17.9536, -45.5906) (-17.9536, -45.2495) knots 0 0 0 1 2 2 2
  spline S158 degree 2 poles (-17.9536, -45.2495) (-17.9536, -44.9084) (-18.275, -44.4685) (-18.5963, -44.34) knots 0 0 0 1 2 2 2
  spline S159 degree 2 poles (-18.5963, -44.34) (-18.9077, -44.2164) (-19.8568, -44.1274) (-20.4549, -44.1274) knots 0 0 0 1 2 2 2
  spline S160 degree 2 poles (-20.4549, -44.1274) (-21.0976, -44.1274) (-21.9577, -44.2065) (-22.2938, -44.335) knots 0 0 0 1 2 2 2
  spline S161 degree 2 poles (-22.2938, -44.335) (-22.6102, -44.4536) (-22.9513, -44.8936) (-22.9513, -45.2495) knots 0 0 0 1 2 2 2
  spline S162 degree 2 poles (-22.9513, -45.2495) (-22.9513, -45.5857) (-22.63, -46.0256) (-22.3087, -46.1492) knots 0 0 0 1 2 2 2
  line L125 (-23.5, -53.2823) -> (-20.8504, -53.2823)
  spline S163 degree 2 poles (-20.8504, -53.2823) (-20.534, -53.2823) (-19.9952, -53.2329) (-19.8469, -53.1538) knots 0 0 0 1 2 2 2
  spline S164 degree 2 poles (-19.8469, -53.1538) (-19.6838, -53.0747) (-19.5256, -52.7732) (-19.5256, -52.5112) knots 0 0 0 1 2 2 2
  spline S165 degree 2 poles (-19.5256, -52.5112) (-19.5256, -52.2739) (-19.8173, -51.7301) (-20.0941, -51.4434) knots 0 0 0 1 2 2 2
  spline S166 degree 2 poles (-20.0941, -51.4434) (-20.1633, -51.4484) (-20.3561, -51.4583) (-20.4846, -51.4583) knots 0 0 0 1 2 2 2
  line L126 (-20.4846, -51.4583) -> (-23.5, -51.4583)
  line L127 (-23.5, -51.4583) -> (-23.5, -50.6871)
  line L128 (-23.5, -50.6871) -> (-20.8504, -50.6871)
  spline S167 degree 2 poles (-20.8504, -50.6871) (-20.534, -50.6871) (-19.9952, -50.6377) (-19.8469, -50.5586) knots 0 0 0 1 2 2 2
  spline S168 degree 2 poles (-19.8469, -50.5586) (-19.6838, -50.4795) (-19.5256, -50.178) (-19.5256, -49.916) knots 0 0 0 1 2 2 2
  spline S169 degree 2 poles (-19.5256, -49.916) (-19.5256, -49.6688) (-19.837, -49.1201) (-20.0793, -48.863) knots 0 0 0 1 2 2 2
  line L129 (-20.0793, -48.863) -> (-23.5, -48.863)
  line L130 (-23.5, -48.863) -> (-23.5, -48.0919)
  line L131 (-23.5, -48.0919) -> (-18.9225, -48.0919)
  line L132 (-18.9225, -48.0919) -> (-18.9225, -48.863)
  line L133 (-18.9225, -48.863) -> (-19.4267, -48.863)
  spline S170 degree 2 poles (-19.4267, -48.863) (-19.1252, -49.1646) (-18.794, -49.7578) (-18.794, -50.1137) knots 0 0 0 1 2 2 2
  spline S171 degree 2 poles (-18.794, -50.1137) (-18.794, -50.519) (-19.1647, -51.1468) (-19.5849, -51.31) knots 0 0 0 1 2 2 2
  spline S172 degree 2 poles (-19.5849, -51.31) (-19.1944, -51.6609) (-18.794, -52.3233) (-18.794, -52.7089) knots 0 0 0 1 2 2 2
  spline S173 degree 2 poles (-18.794, -52.7089) (-18.794, -53.0055) (-18.9769, -53.49) (-19.1845, -53.6679) knots 0 0 0 1 2 2 2
  spline S174 degree 2 poles (-19.1845, -53.6679) (-19.3921, -53.8508) (-20.015, -54.0535) (-20.4846, -54.0535) knots 0 0 0 1 2 2 2
  line L134 (-20.4846, -54.0535) -> (-23.5, -54.0535)
  line L135 (-23.5, -54.0535) -> (-23.5, -53.2823)
  line L136 (-23.5, -60.3265) -> (-20.8504, -60.3265)
  spline S175 degree 2 poles (-20.8504, -60.3265) (-20.534, -60.3265) (-19.9952, -60.2771) (-19.8469, -60.198) knots 0 0 0 1 2 2 2
  spline S176 degree 2 poles (-19.8469, -60.198) (-19.6838, -60.1189) (-19.5256, -59.8173) (-19.5256, -59.5553) knots 0 0 0 1 2 2 2
  spline S177 degree 2 poles (-19.5256, -59.5553) (-19.5256, -59.3181) (-19.8173, -58.7743) (-20.0941, -58.4876) knots 0 0 0 1 2 2 2
  spline S178 degree 2 poles (-20.0941, -58.4876) (-20.1633, -58.4925) (-20.3561, -58.5024) (-20.4846, -58.5024) knots 0 0 0 1 2 2 2
  line L137 (-20.4846, -58.5024) -> (-23.5, -58.5024)
  line L138 (-23.5, -58.5024) -> (-23.5, -57.7313)
  line L139 (-23.5, -57.7313) -> (-20.8504, -57.7313)
  spline S179 degree 2 poles (-20.8504, -57.7313) (-20.534, -57.7313) (-19.9952, -57.6818) (-19.8469, -57.6028) knots 0 0 0 1 2 2 2
  spline S180 degree 2 poles (-19.8469, -57.6028) (-19.6838, -57.5237) (-19.5256, -57.2221) (-19.5256, -56.9601) knots 0 0 0 1 2 2 2
  spline S181 degree 2 poles (-19.5256, -56.9601) (-19.5256, -56.713) (-19.837, -56.1643) (-20.0793, -55.9072) knots 0 0 0 1 2 2 2
  line L140 (-20.0793, -55.9072) -> (-23.5, -55.9072)
  line L141 (-23.5, -55.9072) -> (-23.5, -55.1361)
  line L142 (-23.5, -55.1361) -> (-18.9225, -55.1361)
  line L143 (-18.9225, -55.1361) -> (-18.9225, -55.9072)
  line L144 (-18.9225, -55.9072) -> (-19.4267, -55.9072)
  spline S182 degree 2 poles (-19.4267, -55.9072) (-19.1252, -56.2088) (-18.794, -56.8019) (-18.794, -57.1579) knots 0 0 0 1 2 2 2
  spline S183 degree 2 poles (-18.794, -57.1579) (-18.794, -57.5632) (-19.1647, -58.191) (-19.5849, -58.3541) knots 0 0 0 1 2 2 2
  spline S184 degree 2 poles (-19.5849, -58.3541) (-19.1944, -58.7051) (-18.794, -59.3675) (-18.794, -59.7531) knots 0 0 0 1 2 2 2
  spline S185 degree 2 poles (-18.794, -59.7531) (-18.794, -60.0497) (-18.9769, -60.5341) (-19.1845, -60.7121) knots 0 0 0 1 2 2 2
  spline S186 degree 2 poles (-19.1845, -60.7121) (-19.3921, -60.895) (-20.015, -61.0976) (-20.4846, -61.0976) knots 0 0 0 1 2 2 2
  line L145 (-20.4846, -61.0976) -> (-23.5, -61.0976)
  line L146 (-23.5, -61.0976) -> (-23.5, -60.3265)
  spline S187 degree 2 poles (-31.5227, -42.679) (-31.9923, -42.679) (-32.7882, -42.3676) (-33.0551, -42.1056) knots 0 0 0 1 2 2 2
  spline S188 degree 2 poles (-33.0551, -42.1056) (-33.3369, -41.8337) (-33.6285, -41.1515) (-33.6285, -40.7412) knots 0 0 0 1 2 2 2
  spline S189 degree 2 poles (-33.6285, -40.7412) (-33.6285, -40.331) (-33.3517, -39.6537) (-33.0749, -39.3967) knots 0 0 0 1 2 2 2
  spline S190 degree 2 poles (-33.0749, -39.3967) (-32.7437, -39.0803) (-31.6314, -38.7244) (-30.8207, -38.7244) knots 0 0 0 1 2 2 2
  spline S191 degree 2 poles (-30.8207, -38.7244) (-30.0249, -38.7244) (-28.7446, -39.0506) (-28.27, -39.3917) knots 0 0 0 1 2 2 2
  spline S192 degree 2 poles (-28.27, -39.3917) (-27.8053, -39.7229) (-27.2863, -40.7709) (-27.2863, -41.458) knots 0 0 0 1 2 2 2
  spline S193 degree 2 poles (-27.2863, -41.458) (-27.2863, -41.6607) (-27.3259, -42.0166) (-27.3703, -42.1501) knots 0 0 0 1 2 2 2
  line L147 (-27.3703, -42.1501) -> (-28.1563, -42.1501)
  line L148 (-28.1563, -42.1501) -> (-28.1563, -42.1155)
  spline S194 degree 2 poles (-28.1563, -42.1155) (-28.097, -42.0018) (-27.9932, -41.5865) (-27.9932, -41.3493) knots 0 0 0 1 2 2 2
  spline S195 degree 2 poles (-27.9932, -41.3493) (-27.9932, -40.588) (-29.0214, -39.6537) (-30.0298, -39.5647) knots 0 0 0 1 2 2 2
  spline S196 degree 2 poles (-30.0298, -39.5647) (-29.8271, -39.8564) (-29.6047, -40.4694) (-29.6047, -40.8352) knots 0 0 0 1 2 2 2
  spline S197 degree 2 poles (-29.6047, -40.8352) (-29.6047, -41.1911) (-29.7481, -41.725) (-29.9656, -42.0166) knots 0 0 0 1 2 2 2
  spline S198 degree 2 poles (-29.9656, -42.0166) (-30.2177, -42.3528) (-30.9987, -42.679) (-31.5227, -42.679) knots 0 0 0 1 2 2 2
  spline S199 degree 2 poles (-31.5573, -41.8485) (-31.1816, -41.8485) (-30.6724, -41.6508) (-30.4945, -41.4333) knots 0 0 0 1 2 2 2
  spline S200 degree 2 poles (-30.4945, -41.4333) (-30.366, -41.2702) (-30.2819, -40.8648) (-30.2819, -40.6523) knots 0 0 0 1 2 2 2
  spline S201 degree 2 poles (-30.2819, -40.6523) (-30.2819, -40.3656) (-30.4549, -39.8267) (-30.6181, -39.5647) knots 0 0 0 1 2 2 2
  spline S202 degree 2 poles (-30.6181, -39.5647) (-30.7071, -39.5598) (-30.8751, -39.5499) (-31.0036, -39.5499) knots 0 0 0 1 2 2 2
  spline S203 degree 2 poles (-31.0036, -39.5499) (-31.6364, -39.5499) (-32.4125, -39.7971) (-32.6152, -39.9849) knots 0 0 0 1 2 2 2
  spline S204 degree 2 poles (-32.6152, -39.9849) (-32.8079, -40.1579) (-32.9612, -40.5336) (-32.9612, -40.7462) knots 0 0 0 1 2 2 2
  spline S205 degree 2 poles (-32.9612, -40.7462) (-32.9612, -41.2405) (-32.2592, -41.8485) (-31.5573, -41.8485) knots 0 0 0 1 2 2 2
  spline S206 degree 2 poles (-30.45, -47.1972) (-32.0912, -47.1972) (-33.6285, -46.2431) (-33.6285, -45.2495) knots 0 0 0 1 2 2 2
  spline S207 degree 2 poles (-33.6285, -45.2495) (-33.6285, -44.2411) (-32.0615, -43.2969) (-30.4549, -43.2969) knots 0 0 0 1 2 2 2
  spline S208 degree 2 poles (-30.4549, -43.2969) (-28.8039, -43.2969) (-27.2764, -44.251) (-27.2764, -45.2495) knots 0 0 0 1 2 2 2
  spline S209 degree 2 poles (-27.2764, -45.2495) (-27.2764, -46.253) (-28.8583, -47.1972) (-30.45, -47.1972) knots 0 0 0 1 2 2 2
  spline S210 degree 2 poles (-32.3087, -46.1492) (-32.0071, -46.2678) (-31.0778, -46.3667) (-30.45, -46.3667) knots 0 0 0 1 2 2 2
  spline S211 degree 2 poles (-30.45, -46.3667) (-29.8222, -46.3667) (-28.8978, -46.2678) (-28.5864, -46.1442) knots 0 0 0 1 2 2 2
  spline S212 degree 2 poles (-28.5864, -46.1442) (-28.275, -46.0207) (-27.9536, -45.5906) (-27.9536, -45.2495) knots 0 0 0 1 2 2 2
  spline S213 degree 2 poles (-27.9536, -45.2495) (-27.9536, -44.9084) (-28.275, -44.4685) (-28.5963, -44.34) knots 0 0 0 1 2 2 2
  spline S214 degree 2 poles (-28.5963, -44.34) (-28.9077, -44.2164) (-29.8568, -44.1274) (-30.4549, -44.1274) knots 0 0 0 1 2 2 2
  spline S215 degree 2 poles (-30.4549, -44.1274) (-31.0976, -44.1274) (-31.9577, -44.2065) (-32.2938, -44.335) knots 0 0 0 1 2 2 2
  spline S216 degree 2 poles (-32.2938, -44.335) (-32.6102, -44.4536) (-32.9513, -44.8936) (-32.9513, -45.2495) knots 0 0 0 1 2 2 2
  spline S217 degree 2 poles (-32.9513, -45.2495) (-32.9513, -45.5857) (-32.63, -46.0256) (-32.3087, -46.1492) knots 0 0 0 1 2 2 2
  line L149 (-33.5, -53.2823) -> (-30.8504, -53.2823)
  spline S218 degree 2 poles (-30.8504, -53.2823) (-30.534, -53.2823) (-29.9952, -53.2329) (-29.8469, -53.1538) knots 0 0 0 1 2 2 2
  spline S219 degree 2 poles (-29.8469, -53.1538) (-29.6838, -53.0747) (-29.5256, -52.7732) (-29.5256, -52.5112) knots 0 0 0 1 2 2 2
  spline S220 degree 2 poles (-29.5256, -52.5112) (-29.5256, -52.2739) (-29.8173, -51.7301) (-30.0941, -51.4434) knots 0 0 0 1 2 2 2
  spline S221 degree 2 poles (-30.0941, -51.4434) (-30.1633, -51.4484) (-30.3561, -51.4583) (-30.4846, -51.4583) knots 0 0 0 1 2 2 2
  line L150 (-30.4846, -51.4583) -> (-33.5, -51.4583)
  line L151 (-33.5, -51.4583) -> (-33.5, -50.6871)
  line L152 (-33.5, -50.6871) -> (-30.8504, -50.6871)
  spline S222 degree 2 poles (-30.8504, -50.6871) (-30.534, -50.6871) (-29.9952, -50.6377) (-29.8469, -50.5586) knots 0 0 0 1 2 2 2
  spline S223 degree 2 poles (-29.8469, -50.5586) (-29.6838, -50.4795) (-29.5256, -50.178) (-29.5256, -49.916) knots 0 0 0 1 2 2 2
  spline S224 degree 2 poles (-29.5256, -49.916) (-29.5256, -49.6688) (-29.837, -49.1201) (-30.0793, -48.863) knots 0 0 0 1 2 2 2
  line L153 (-30.0793, -48.863) -> (-33.5, -48.863)
  line L154 (-33.5, -48.863) -> (-33.5, -48.0919)
  line L155 (-33.5, -48.0919) -> (-28.9225, -48.0919)
  line L156 (-28.9225, -48.0919) -> (-28.9225, -48.863)
  line L157 (-28.9225, -48.863) -> (-29.4267, -48.863)
  spline S225 degree 2 poles (-29.4267, -48.863) (-29.1252, -49.1646) (-28.794, -49.7578) (-28.794, -50.1137) knots 0 0 0 1 2 2 2
  spline S226 degree 2 poles (-28.794, -50.1137) (-28.794, -50.519) (-29.1647, -51.1468) (-29.5849, -51.31) knots 0 0 0 1 2 2 2
  spline S227 degree 2 poles (-29.5849, -51.31) (-29.1944, -51.6609) (-28.794, -52.3233) (-28.794, -52.7089) knots 0 0 0 1 2 2 2
  spline S228 degree 2 poles (-28.794, -52.7089) (-28.794, -53.0055) (-28.9769, -53.49) (-29.1845, -53.6679) knots 0 0 0 1 2 2 2
  spline S229 degree 2 poles (-29.1845, -53.6679) (-29.3921, -53.8508) (-30.015, -54.0535) (-30.4846, -54.0535) knots 0 0 0 1 2 2 2
  line L158 (-30.4846, -54.0535) -> (-33.5, -54.0535)
  line L159 (-33.5, -54.0535) -> (-33.5, -53.2823)
  line L160 (-33.5, -60.3265) -> (-30.8504, -60.3265)
  spline S230 degree 2 poles (-30.8504, -60.3265) (-30.534, -60.3265) (-29.9952, -60.2771) (-29.8469, -60.198) knots 0 0 0 1 2 2 2
  spline S231 degree 2 poles (-29.8469, -60.198) (-29.6838, -60.1189) (-29.5256, -59.8173) (-29.5256, -59.5553) knots 0 0 0 1 2 2 2
  spline S232 degree 2 poles (-29.5256, -59.5553) (-29.5256, -59.3181) (-29.8173, -58.7743) (-30.0941, -58.4876) knots 0 0 0 1 2 2 2
  spline S233 degree 2 poles (-30.0941, -58.4876) (-30.1633, -58.4925) (-30.3561, -58.5024) (-30.4846, -58.5024) knots 0 0 0 1 2 2 2
  line L161 (-30.4846, -58.5024) -> (-33.5, -58.5024)
  line L162 (-33.5, -58.5024) -> (-33.5, -57.7313)
  line L163 (-33.5, -57.7313) -> (-30.8504, -57.7313)
  spline S234 degree 2 poles (-30.8504, -57.7313) (-30.534, -57.7313) (-29.9952, -57.6818) (-29.8469, -57.6028) knots 0 0 0 1 2 2 2
  spline S235 degree 2 poles (-29.8469, -57.6028) (-29.6838, -57.5237) (-29.5256, -57.2221) (-29.5256, -56.9601) knots 0 0 0 1 2 2 2
  spline S236 degree 2 poles (-29.5256, -56.9601) (-29.5256, -56.713) (-29.837, -56.1643) (-30.0793, -55.9072) knots 0 0 0 1 2 2 2
  line L164 (-30.0793, -55.9072) -> (-33.5, -55.9072)
  line L165 (-33.5, -55.9072) -> (-33.5, -55.1361)
  line L166 (-33.5, -55.1361) -> (-28.9225, -55.1361)
  line L167 (-28.9225, -55.1361) -> (-28.9225, -55.9072)
  line L168 (-28.9225, -55.9072) -> (-29.4267, -55.9072)
  spline S237 degree 2 poles (-29.4267, -55.9072) (-29.1252, -56.2088) (-28.794, -56.8019) (-28.794, -57.1579) knots 0 0 0 1 2 2 2
  spline S238 degree 2 poles (-28.794, -57.1579) (-28.794, -57.5632) (-29.1647, -58.191) (-29.5849, -58.3541) knots 0 0 0 1 2 2 2
  spline S239 degree 2 poles (-29.5849, -58.3541) (-29.1944, -58.7051) (-28.794, -59.3675) (-28.794, -59.7531) knots 0 0 0 1 2 2 2
  spline S240 degree 2 poles (-28.794, -59.7531) (-28.794, -60.0497) (-28.9769, -60.5341) (-29.1845, -60.7121) knots 0 0 0 1 2 2 2
  spline S241 degree 2 poles (-29.1845, -60.7121) (-29.3921, -60.895) (-30.015, -61.0976) (-30.4846, -61.0976) knots 0 0 0 1 2 2 2
  line L169 (-30.4846, -61.0976) -> (-33.5, -61.0976)
  line L170 (-33.5, -61.0976) -> (-33.5, -60.3265)
  line L171 (-38.3145, -42.6543) -> (-43.5, -40.0146)
  line L172 (-43.5, -40.0146) -> (-43.5, -39.1446)
  line L173 (-43.5, -39.1446) -> (-38.1168, -41.9326)
  line L174 (-38.1168, -41.9326) -> (-38.1168, -38.7837)
  line L175 (-38.1168, -38.7837) -> (-37.4, -38.7837)
  line L176 (-37.4, -38.7837) -> (-37.4, -42.6543)
  line L177 (-37.4, -42.6543) -> (-38.3145, -42.6543)
  spline S242 degree 2 poles (-40.45, -47.1972) (-42.0912, -47.1972) (-43.6285, -46.2431) (-43.6285, -45.2495) knots 0 0 0 1 2 2 2
  spline S243 degree 2 poles (-43.6285, -45.2495) (-43.6285, -44.2411) (-42.0615, -43.2969) (-40.4549, -43.2969) knots 0 0 0 1 2 2 2
  spline S244 degree 2 poles (-40.4549, -43.2969) (-38.8039, -43.2969) (-37.2764, -44.251) (-37.2764, -45.2495) knots 0 0 0 1 2 2 2
  spline S245 degree 2 poles (-37.2764, -45.2495) (-37.2764, -46.253) (-38.8583, -47.1972) (-40.45, -47.1972) knots 0 0 0 1 2 2 2
  spline S246 degree 2 poles (-42.3087, -46.1492) (-42.0071, -46.2678) (-41.0778, -46.3667) (-40.45, -46.3667) knots 0 0 0 1 2 2 2
  spline S247 degree 2 poles (-40.45, -46.3667) (-39.8222, -46.3667) (-38.8978, -46.2678) (-38.5864, -46.1442) knots 0 0 0 1 2 2 2
  spline S248 degree 2 poles (-38.5864, -46.1442) (-38.275, -46.0207) (-37.9536, -45.5906) (-37.9536, -45.2495) knots 0 0 0 1 2 2 2
  spline S249 degree 2 poles (-37.9536, -45.2495) (-37.9536, -44.9084) (-38.275, -44.4685) (-38.5963, -44.34) knots 0 0 0 1 2 2 2
  spline S250 degree 2 poles (-38.5963, -44.34) (-38.9077, -44.2164) (-39.8568, -44.1274) (-40.4549, -44.1274) knots 0 0 0 1 2 2 2
  spline S251 degree 2 poles (-40.4549, -44.1274) (-41.0976, -44.1274) (-41.9577, -44.2065) (-42.2938, -44.335) knots 0 0 0 1 2 2 2
  spline S252 degree 2 poles (-42.2938, -44.335) (-42.6102, -44.4536) (-42.9513, -44.8936) (-42.9513, -45.2495) knots 0 0 0 1 2 2 2
  spline S253 degree 2 poles (-42.9513, -45.2495) (-42.9513, -45.5857) (-42.63, -46.0256) (-42.3087, -46.1492) knots 0 0 0 1 2 2 2
  line L178 (-43.5, -53.2823) -> (-40.8504, -53.2823)
  spline S254 degree 2 poles (-40.8504, -53.2823) (-40.534, -53.2823) (-39.9952, -53.2329) (-39.8469, -53.1538) knots 0 0 0 1 2 2 2
  spline S255 degree 2 poles (-39.8469, -53.1538) (-39.6838, -53.0747) (-39.5256, -52.7732) (-39.5256, -52.5112) knots 0 0 0 1 2 2 2
  spline S256 degree 2 poles (-39.5256, -52.5112) (-39.5256, -52.2739) (-39.8173, -51.7301) (-40.0941, -51.4434) knots 0 0 0 1 2 2 2
  spline S257 degree 2 poles (-40.0941, -51.4434) (-40.1633, -51.4484) (-40.3561, -51.4583) (-40.4846, -51.4583) knots 0 0 0 1 2 2 2
  line L179 (-40.4846, -51.4583) -> (-43.5, -51.4583)
  line L180 (-43.5, -51.4583) -> (-43.5, -50.6871)
  line L181 (-43.5, -50.6871) -> (-40.8504, -50.6871)
  spline S258 degree 2 poles (-40.8504, -50.6871) (-40.534, -50.6871) (-39.9952, -50.6377) (-39.8469, -50.5586) knots 0 0 0 1 2 2 2
  spline S259 degree 2 poles (-39.8469, -50.5586) (-39.6838, -50.4795) (-39.5256, -50.178) (-39.5256, -49.916) knots 0 0 0 1 2 2 2
  spline S260 degree 2 poles (-39.5256, -49.916) (-39.5256, -49.6688) (-39.837, -49.1201) (-40.0793, -48.863) knots 0 0 0 1 2 2 2
  line L182 (-40.0793, -48.863) -> (-43.5, -48.863)
  line L183 (-43.5, -48.863) -> (-43.5, -48.0919)
  line L184 (-43.5, -48.0919) -> (-38.9225, -48.0919)
  line L185 (-38.9225, -48.0919) -> (-38.9225, -48.863)
  line L186 (-38.9225, -48.863) -> (-39.4267, -48.863)
  spline S261 degree 2 poles (-39.4267, -48.863) (-39.1252, -49.1646) (-38.794, -49.7578) (-38.794, -50.1137) knots 0 0 0 1 2 2 2
  spline S262 degree 2 poles (-38.794, -50.1137) (-38.794, -50.519) (-39.1647, -51.1468) (-39.5849, -51.31) knots 0 0 0 1 2 2 2